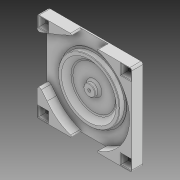
# Autodesk Inventor part: Base
Saved by Autodesk Inventor 2020 (Build 240168000, 168)
## iProperties
Created: 2020-10-19
Part Number: Base
Material: Generic
Document SubType Name: Modeling
Designer: DDeGo
Density: 1 g/cm^3
Appearance: Default
Author: DDeGo
Autodesk Inventor part; units mm, degrees
ref_plane "YZ Plane" through (0, 0, 0) normal (1, 0, 0) x (0, 1, 0)
ref_plane "XZ Plane" through (0, 0, 0) normal (0, 1, 0) x (-1, 0, 0)
sketch "Sketch1" plane through (0, 0, 0) normal (0, 0, 1) x (1, 0, 0)
  line L0 (-97.5, -92.5) -> (97.5, -92.5)
  line L1 (97.5, -92.5) -> (97.5, 92.5)
  line L2 (97.5, 92.5) -> (-97.5, 92.5)
  line L3 (-97.5, 92.5) -> (-97.5, -92.5)
  line L4 (-97.5, -92.5) -> (97.5, 92.5) construction
  line L5 (97.5, -92.5) -> (-97.5, 92.5) construction
  circle A0 centre (0, 0) radius 90 construction
  dimension "d0" = 185
  dimension "d2" = 180
  dimension "d22" = 195
  constraints: 12 end point, 2 midpoint, 2 parallel, 1 centre point, 1 coincident, 1 horizontal, 1 perpendicular
  measures "d0" distance of L0.end L1.end
  measures "d2" diameter of A0
  measures "d22" distance of L1.end L2.end
extrude "Extrusion1" add sketch "Sketch1" along normal blind 3
sketch "Sketch2" plane through (0, 0, 3) normal (0, 0, 1) x (1, 0, 0)
  line L0 (-97.5, 92.5) -> (-97.5, -92.5) projected
  line L1 (-97.5, -92.5) -> (97.5, -92.5) projected
  line L2 (97.5, -92.5) -> (97.5, 92.5) projected
  line L3 (97.5, 92.5) -> (-97.5, 92.5) projected
  circle A0 centre (0, 0) radius 93
  circle A1 centre (0, 0) radius 90 construction
  point P0 (92.5, -21.6506)
  point P1 (9.6307, -92.5)
  point P2 (-9.6307, -92.5)
  point P3 (-92.5, -21.6506)
  point P4 (9.6307, 92.5)
  point P5 (92.5, 21.6506)
  point P6 (-92.5, 21.6506)
  point P7 (-9.6307, 92.5)
  dimension "d5" = 180
  dimension "d6" = 3
  constraints: 2 centre point, 2 coincident
  measures "d5" diameter of A1
  measures "d6" radial gap between concentric circles of A0 A1
extrude "Extrusion2" add sketch "Sketch2" along normal blind 20 contours L3 A0 L1 L0 | L3 L2 L1 A0
sketch "Sketch3" plane through (0, 0, 23) normal (0, 0, 1) x (1, 0, 0)
  line L0 (-95.15, -90.15) -> (-74.85, -90.15)
  line L1 (-74.85, -90.15) -> (-74.85, -69.85)
  line L2 (-74.85, -69.85) -> (-95.15, -69.85)
  line L3 (-95.15, -69.85) -> (-95.15, -90.15)
  line L4 (-95.15, -90.15) -> (-74.85, -69.85) construction
  line L5 (-74.85, -90.15) -> (-95.15, -69.85) construction
  line L6 (85, 80) -> (-85, 80) construction
  line L7 (-85, 80) -> (-85, -80) construction
  line L8 (-85, -80) -> (85, -80) construction
  line L9 (85, -80) -> (85, 80) construction
  line L10 (85, 80) -> (-85, -80) construction
  line L11 (-85, 80) -> (85, -80) construction
  point P0 (0, 0)
  dimension "d9" = 20.3
  dimension "d10" = 20.3
  dimension "d11" = 160
  dimension "d12" = 170
  constraints: 24 end point, 4 midpoint, 4 parallel, 2 horizontal, 2 perpendicular
  measures "d9" distance of L1.end L2.end
  measures "d10" distance of L0.end L1.end
  measures "d11" distance of L8.end L6.start
  measures "d12" distance of L7.end L8.end
ref_plane "Work Plane1" through (0, 0, 7.5) normal (0, 0, -1) x (-1, 0, 0)
extrude "Extrusion3" cut sketch "Sketch3" against normal up to surface (15.5 mm away)
sketch "Sketch4" plane through (-95.15, -90.15, 7.5) normal (0, 0, 1) x (1, 0, 0)
  line L0 (20.3, 20.3) -> (20.3, 0) projected
  line L1 (0, 20.3) -> (20.3, 0) construction
  circle A0 centre (10.15, 10.15) radius 3
  point P0 (95.15, 90.15)
  dimension "d16" = 6
  constraints: 2 end point, 1 centre point, 1 midpoint
  measures "d16" diameter of A0
extrude "Extrusion4" cut sketch "Sketch4" against normal blind 15
mirror "Mirror1" about plane through (0, 0, 0) normal (0, 1, 0) of "Extrusion3", "Extrusion4"
mirror "Mirror2" about plane through (0, 0, 0) normal (1, 0, 0) of "Extrusion3", "Extrusion4", "Mirror1"
sketch "Sketch5" plane through (0, 0, 0) normal (0, 1, 0) x (-1, 0, 0)
  line L0 (-9.6307, 3) -> (9.6307, 3) construction
  line L1 (0, 3) -> (56.35, 3) construction
  line L2 (67.35, 3) -> (67.35, 4)
  line L3 (67.35, 4) -> (63.35, 4)
  line L4 (63.35, 4) -> (63.35, 14)
  line L5 (63.35, 14) -> (56.35, 14)
  line L6 (56.35, 14) -> (56.35, 3) construction
  line L7 (56.35, 3) -> (67.35, 3)
  line L8 (0, 3) -> (0, 13)
  line L9 (56.35, 3) -> (45.35, 3)
  line L10 (56.35, 14) -> (45.35, 3)
  line L11 (0, 13) -> (12, 13)
  line L12 (12, 13) -> (12, 3)
  line L13 (12, 3) -> (0, 3)
  point P0 (0, 0)
  dimension "d23" = 63.35
  dimension "d24" = 4
  dimension "d25" = 1
  dimension "d26" = 10
  dimension "d27" = 7
  dimension "d28" = 45
  dimension "d54" = 10
  dimension "d55" = 12
  constraints: 26 end point, 9 perpendicular, 3 horizontal, 2 point on line, 1 midpoint, 1 vertical
  measures "d23" distance between parallel lines of L8 L4
  measures "d24" distance of L2.end L3.end
  measures "d25" distance of L2.start L2.end
  measures "d26" distance of L3.end L4.end
  measures "d27" distance of L4.end L5.end
  measures "d28" angle of L6 L10
  measures "d54" distance of L11.end L12.end
  measures "d55" distance of L8.end L11.end
revolve "Revolution1" add sketch "Sketch5" angle 360 about axis through (0, 0, 3) along (0, 0, 1)
chamfer "Chamfer1" distance 1 angle 45 1 edges at (63.35, 0, 14)
sketch "Sketch6" plane through (0, 0, 23) normal (0, 0, 1) x (1, 0, 0)
  line L0 (-46.5698, 80.5) -> (-97.5, 60.5)
  line L1 (-97.5, 60.5) -> (-97.5, -27.5)
  line L2 (-97.5, -27.5) -> (-76.7642, -52.5)
  line L3 (-97.5, 92.5) -> (-97.5, -92.5) projected
  arc A0 (-9.6307, 92.5) -> (-9.6307, -92.5) centre (0, 0) ccw projected
  line L4 (-9.6307, 92.5) -> (-97.5, 92.5) projected
  dimension "d33" = 32
  dimension "d34" = 12
  dimension "d35" = 120
  dimension "d36" = 25
  constraints: 6 end point, 2 point on circle, 1 point on line, 1 vertical
  measures "d33" distance of L3.start L0.end
  measures "d34" distance from line of L4 L0.start
  measures "d35" distance from line of L4 L1.end
  measures "d36" vertical distance of L1.end L2.end
extrude "Extrusion5" cut sketch "Sketch6" against normal up to surface (20 mm away) contours A0 L2 L1 L0
fillet "Fillet1" radius 5 2 edges at (-97.5, 60.5, 13) (-97.5, -27.5, 13)
fillet "Fillet1" radius 2 4 edges at (9.6307, 92.5, 13) (-9.6307, 92.5, 13) (-9.6307, -92.5, 13) (9.6307, -92.5, 13)
fillet "Fillet2" radius 4 4 edges at (97.5, 92.5, 11.5) (-97.5, 92.5, 11.5) (97.5, -92.5, 11.5) (-97.5, -92.5, 11.5)
chamfer "Chamfer2" distance 1 angle 45 16 edges at (85, 69.85, 23) (95.15, 80, 23) (74.85, 80, 23) (85, 90.15, 23) (-85, 69.85, 23) (-95.15, 80, 23) (-74.85, 80, 23) (-85, 90.15, 23) (-85, -69.85, 23) (-74.85, -80, 23) (-85, -90.15, 23) (-95.15, -80, 23) (85, -90.15, 23) (95.15, -80, 23) (74.85, -80, 23) (85, -69.85, 23)
sketch "Sketch7" plane through (0, 0, 0) normal (0, 0, -1) x (-1, 0, 0)
  circle A0 centre (-85, 80) radius 3 projected
  circle A1 centre (-85, 80) radius 4.5
  circle A2 centre (-85, -80) radius 3 projected
  circle A3 centre (-85, -80) radius 4.5
  circle A4 centre (85, -80) radius 3 projected
  circle A5 centre (85, -80) radius 4.5
  circle A6 centre (85, 80) radius 3 projected
  circle A7 centre (85, 80) radius 4.5
  point P0 (0, 0)
  dimension "d45" = 9
  constraints: 4 centre point, 4 coincident, 3 equal radius
  measures "d45" diameter of A1
extrude "Extrusion6" cut sketch "Sketch7" against normal blind 5 contours A0 | A1 | A2 | A3 | A4 | A5 | A6 | A7
sketch "Sketch8" plane through (0, 0, 0) normal (0, 0, -1) x (-1, 0, 0)
  line L0 (-75, -70) -> (75, -70) construction
  line L1 (75, -70) -> (75, 70) construction
  line L2 (75, 70) -> (-75, 70) construction
  line L3 (-75, 70) -> (-75, -70) construction
  line L4 (-75, -70) -> (75, 70) construction
  line L5 (75, -70) -> (-75, 70) construction
  circle A0 centre (-75, 70) radius 6
  circle A1 centre (75, 70) radius 6
  circle A2 centre (-75, -70) radius 6
  circle A3 centre (75, -70) radius 6
  line L6 (-93.5, 92.5) -> (93.5, 92.5) projected
  line L7 (-97.5, -88.5) -> (-97.5, 88.5) projected
  point P0 (0, 0)
  dimension "d49" = 12
  dimension "d52" = 22.5
  dimension "d53" = 22.5
  constraints: 12 end point, 4 centre point, 4 coincident, 3 equal radius, 2 midpoint, 2 parallel, 1 horizontal, 1 perpendicular
  measures "d49" diameter of A0
  measures "d52" distance between parallel lines of L6 L2
  measures "d53" distance between parallel lines of L7 L3
extrude "Extrusion7" cut sketch "Sketch8" against normal blind 2.5
sketch "Sketch9" plane through (0, 0, 0) normal (0, 1, 0) x (-1, 0, 0)
  line L0 (0, 0) -> (0, 13)
  line L1 (0, 13) -> (3, 13)
  line L2 (3, 13) -> (3, 9.3)
  line L3 (3, 9.3) -> (8.15, 9.3)
  line L4 (8.15, 9.3) -> (8.15, 6)
  line L5 (8.15, 5) -> (9.15, 5) construction
  line L6 (9.15, 5) -> (9.15, 0)
  line L7 (-12, 3) -> (12, 3) construction
  line L8 (9.15, 0) -> (0, 0)
  line L9 (-12, 13) -> (12, 13) construction
  line L10 (9.15, 5) -> (8.15, 6)
  line L11 (8.15, 6) -> (8.15, 5) construction
  dimension "d56" = 3
  dimension "d57" = 8.15
  dimension "d58" = 4.3
  dimension "d59" = 9.15
  dimension "d61" = 5
  dimension "d63" = 45
  constraints: 20 end point, 8 perpendicular, 1 horizontal, 1 midpoint, 1 vertical
  measures "d56" distance between parallel lines of L0 L2
  measures "d57" distance between parallel lines of L0 L4
  measures "d58" distance of L3.end L5.start
  measures "d59" distance between parallel lines of L0 L6
  measures "d61" distance of L5.end L6.end
  measures "d63" angle of L5 L10
revolve "Revolution2" cut sketch "Sketch9" angle 360 about axis through (0, 0, 0) along (0, 0, 1)
fillet "Fillet3" radius 4 2 edges at (45.35, 0, 3) (12, 0, 3)
chamfer "Chamfer3" distance 1 angle 45 1 edges at (12, 0, 13)
ref_plane "Work Plane2" through (0, 0, 0) normal (0, 1, 0) x (-1, 0, 0)
ref_plane "Work Plane3" through (0, 0, 0) normal (0, -1, 0) x (1, 0, 0)
ref_plane "Work Plane4" through (0, 0, 0) normal (0, -1, 0) x (1, 0, 0)
equation "\"d52\" = d53"
body "Solid1"
